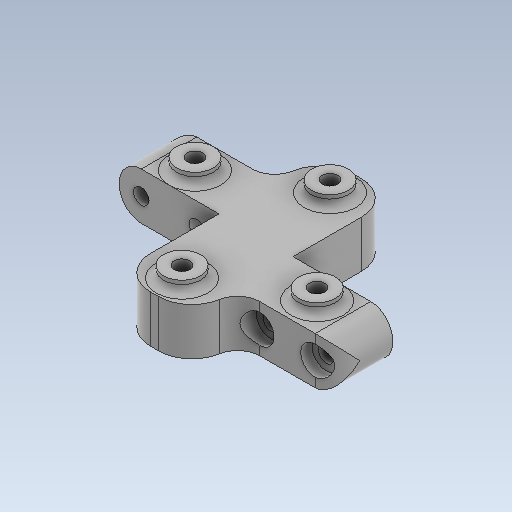
# Autodesk Inventor part: motor_mount
Saved by Autodesk Inventor 2021 (Build 250183000, 183)
## iProperties
Created: 2021-01-21
Part Number: motor_mount
Material: PC/ABS 플라스틱
Document SubType Name: Modeling
Designer: leejun
Density: 0.357273 g/cm^3
Appearance: 매끄러움 - 중간 회색
Author: leejun
Autodesk Inventor part; units mm, degrees
ref_plane "YZ Plane" through (0, 0, 0) normal (1, 0, 0) x (0, 1, 0)
ref_plane "XZ Plane" through (0, 0, 0) normal (0, 1, 0) x (-1, 0, 0)
ref_plane "XY Plane" through (0, 0, 0) normal (0, 0, 1) x (1, 0, 0)
sketch "스케치1" plane through (0, 0, 0) normal (0, 1, 0) x (-1, 0, 0)
  line L0 (-90, -12.7) -> (-10, -12.7) construction
  line L1 (-10, -12.7) -> (-10, 0) construction
  line L2 (-10, 0) -> (-90, 0) construction
  line L3 (-90, 0) -> (-90, -12.7) construction
  line L4 (10, 0) -> (90, 0) construction
  line L5 (90, 0) -> (90, 12.7) construction
  line L6 (90, 12.7) -> (10, 12.7) construction
  line L7 (10, 12.7) -> (10, 0) construction
  line L8 (126, 0) -> (-126, 0) projected
  line L9 (0, -38.5) -> (0, 38.5) projected
  line L10 (-37, 15) -> (10, 15)
  line L11 (10, 15) -> (10, 0)
  line L12 (10, 0) -> (-37, 0)
  line L13 (-37, 0) -> (-37, 15)
  line L14 (37, -15) -> (-10, -15)
  line L15 (-10, -15) -> (-10, 0)
  line L16 (-10, 0) -> (37, 0)
  line L17 (37, 0) -> (37, -15)
  line L18 (-10, -27.5) -> (10, -27.5)
  line L19 (10, -27.5) -> (10, 27.5)
  line L20 (10, 27.5) -> (-10, 27.5)
  line L21 (-10, 27.5) -> (-10, -27.5)
  point P0 (10, 15)
  point P1 (-10, 15)
  point P2 (-37, 0)
  point P3 (10, -15)
  point P4 (37, 0)
  dimension "d68" = 12.7
  dimension "d69" = 80
  dimension "d70" = 20
  dimension "d71" = 27
  dimension "d72" = 15
  dimension "d73" = 55
  constraints: 40 end point, 14 parallel, 7 collinear, 5 perpendicular, 4 horizontal, 3 other
  measures "d68" distance of L0.end L1.end
  measures "d69" distance of L0.start L0.end
  measures "d70" distance between parallel lines of L7 L1
  measures "d71" distance between parallel lines of L17 L7
  measures "d72" distance of L16.end L14.start
  measures "d73" distance of L18.end L19.end
extrude "돌출1" add sketch "스케치1" along normal blind 12.7
sketch "스케치5" plane through (37, 0, 0) normal (0, 0, -1) x (-1, 0, 0)
  line L0 (0, 0) -> (27, 0) projected
  line L1 (27, 0) -> (27, 12.7) projected
  line L2 (0, 12.7) -> (27, 12.7) projected
  line L3 (0, 0) -> (0, 12.7) projected
  circle A0 centre (6, 6.35) radius 6.35
  circle A1 centre (21, 6.35) radius 2.1
  circle A2 centre (6, 6.35) radius 2.1
  line L4 (0, 0) -> (27, 0) projected
  point P0 (37, 0)
  dimension "d74" = 4.2
  dimension "d75" = 6
  dimension "d76" = 15
  constraints: 3 centre point, 2 tangent, 1 coincident, 1 equal radius, 1 horizontal alignment
  measures "d74" diameter of A2
  measures "d75" distance from line of L1 A1.centre
  measures "d76" distance of A1.centre A0.centre
extrude "돌출6" cut sketch "스케치5" against normal through all contours A1 | A2
sketch "스케치6" plane through (10, 0, 15) normal (0, 0, 1) x (1, 0, 0)
  circle A0 centre (6, 6.35) radius 2.1 projected
  circle A1 centre (21, 6.35) radius 2.1 projected
  line L0 (0, 0) -> (27, 0) projected
  line L1 (27, 0) -> (27, 12.7) projected
  line L2 (0, 12.7) -> (27, 12.7) projected
  line L3 (0, 0) -> (0, 12.7) projected
  circle A2 centre (6, 6.35) radius 3.9
  circle A3 centre (21, 6.35) radius 3.9
  point P0 (-10, 0)
  dimension "d82" = 7.8
  constraints: 2 centre point, 2 coincident, 1 equal radius
  measures "d82" diameter of A2
extrude "돌출7" cut sketch "스케치6" against normal blind 3 contours A2 | A3
pattern_circular "원형 패턴3" count 2 over 360 about axis through (0, -10, 0) along (0, 1, 0) of "돌출6", "돌출7"
sketch "스케치7" plane through (0, 12.7, 0) normal (0, 1, 0) x (1, 0, 0)
  line L0 (13.9, -12) -> (18.1, -12) projected
  line L1 (13.9, 0) -> (18.1, 0) projected
  line L2 (28.9, -12) -> (33.1, -12) projected
  line L3 (28.9, 0) -> (33.1, 0) projected
  line L4 (-18.1, 12) -> (-13.9, 12) projected
  line L5 (-13.9, 0) -> (-18.1, 0) projected
  line L6 (-19.9, 12) -> (-12.1, 12) projected
  line L7 (-19.9, 15) -> (-12.1, 15) projected
  line L8 (-33.1, 12) -> (-28.9, 12) projected
  line L9 (-28.9, 0) -> (-33.1, 0) projected
  line L10 (-34.9, 12) -> (-27.1, 12) projected
  line L11 (-34.9, 15) -> (-27.1, 15) projected
  line L12 (19.9, -12) -> (12.1, -12) projected
  line L13 (19.9, -15) -> (12.1, -15) projected
  line L14 (34.9, -12) -> (27.1, -12) projected
  line L15 (34.9, -15) -> (27.1, -15) projected
  line L16 (19.9, -15) -> (12.1, -15) projected
  line L17 (12.1, -15) -> (12.1, -12)
  line L18 (13.9, 0) -> (18.1, 0) projected
  line L19 (13.9, 0) -> (13.9, -12)
  line L20 (13.9, 0) -> (13.9, -12) projected
  line L21 (18.1, 0) -> (18.1, -12)
  line L22 (18.1, 0) -> (18.1, -12) projected
  line L23 (19.9, -12) -> (12.1, -12) projected
  line L24 (19.9, -12) -> (19.9, -15)
  line L25 (19.9, -15) -> (19.9, -12) projected
  line L26 (34.9, -15) -> (27.1, -15) projected
  line L27 (27.1, -15) -> (27.1, -12)
  line L28 (27.1, -15) -> (27.1, -12) projected
  line L29 (34.9, -12) -> (27.1, -12) projected
  line L30 (34.9, -12) -> (34.9, -15)
  line L31 (34.9, -15) -> (34.9, -12) projected
  line L32 (28.9, -12) -> (33.1, -12) projected
  line L33 (28.9, 0) -> (28.9, -12)
  line L34 (33.1, 0) -> (33.1, -12)
  line L35 (37, 0) -> (10, 0) projected
  line L36 (-13.9, 0) -> (-18.1, 0) projected
  line L37 (-18.1, 0) -> (-18.1, 12)
  line L38 (-18.1, 0) -> (-18.1, 12) projected
  line L39 (-19.9, 12) -> (-12.1, 12) projected
  line L40 (-19.9, 12) -> (-19.9, 15)
  line L41 (-19.9, 15) -> (-19.9, 12) projected
  line L42 (-12.1, 15) -> (-12.1, 12)
  line L43 (-12.1, 15) -> (-12.1, 12) projected
  line L44 (-13.9, 0) -> (-13.9, 12)
  line L45 (-13.9, 0) -> (-13.9, 12) projected
  line L46 (-33.1, 12) -> (-28.9, 12) projected
  line L47 (-28.9, 0) -> (-28.9, 12)
  line L48 (-33.1, 0) -> (-33.1, 12)
  line L49 (-37, 0) -> (-10, 0) projected
  line L50 (-34.9, 12) -> (-34.9, 15)
  line L51 (-27.1, 15) -> (-27.1, 12)
  line L52 (-27.1, 15) -> (-27.1, 12) projected
  line L53 (-10, -27.5) -> (10, -27.5) projected
  line L54 (10, -27.5) -> (10, -15) projected
  line L55 (10, -15) -> (37, -15) projected
  line L56 (37, -15) -> (37, 0) projected
  line L57 (37, 0) -> (10, 0) projected
  line L58 (10, 0) -> (10, 27.5) projected
  line L59 (10, 27.5) -> (-10, 27.5) projected
  line L60 (-10, 27.5) -> (-10, 15) projected
  line L61 (-10, 15) -> (-37, 15) projected
  line L62 (-37, 15) -> (-37, 0) projected
  line L63 (-37, 0) -> (-10, 0) projected
  line L64 (-10, 0) -> (-10, -27.5) projected
  circle A0 centre (0, -20) radius 2.1
  circle A1 centre (0, 20) radius 2.1
  circle A2 centre (23.5, -7) radius 2.1
  circle A3 centre (-23.5, 7) radius 2.1
  line L65 (0, 38.5) -> (0, -38.5) projected
  line L66 (-51.8, 0) -> (51.8, 0) projected
  line L67 (23.5, -7) -> (-23.5, -7) construction
  line L68 (-23.5, -7) -> (-23.5, 7) construction
  line L69 (-23.5, 7) -> (23.5, 7) construction
  line L70 (23.5, 7) -> (23.5, -7) construction
  point P0 (0, 0)
  dimension "d85" = 4.2
  dimension "d86" = 20
  dimension "d87" = 5.4
  dimension "d88" = 5.4
  dimension "d89" = 7
  constraints: 40 end point, 10 collinear, 4 centre point, 4 equal radius, 4 parallel, 4 perpendicular, 2 vertical, 1 horizontal, 1 point on line, 2 other
  measures "d85" diameter of A3
  measures "d87" distance between parallel lines of L21 L70
  measures "d88" distance between parallel lines of L33 L70
  measures "d89" distance of the line from the sketch origin of L67
extrude "돌출8" cut sketch "스케치7" against normal through all contours L65 A1 | A1 L65 | L65 A0 | A0 L65 | A2 | A3
fillet "모깎기4" radius 6 4 edges at (37, 6.35, 15) (10, 6.35, 15) (-10, 6.35, -15) (-37, 6.35, -15)
fillet "모깎기4" radius 9 4 edges at (-10, 6.35, -27.5) (10, 6.35, -27.5) (10, 6.35, 27.5) (-10, 6.35, 27.5)
sketch "스케치8" plane through (0, 12.7, 0) normal (0, 1, 0) x (1, 0, 0)
  arc A0 (-31, 15) -> (-37, 9) centre (-31, 9) ccw projected
  line L0 (-37, 9) -> (-37, 0) projected
  line L1 (-37, 0) -> (-10, 0) projected
  line L2 (-10, 0) -> (-10, -18.5) projected
  arc A1 (-10, -18.5) -> (-1, -27.5) centre (-1, -18.5) ccw projected
  line L3 (-1, -27.5) -> (1.2098, -27.5) projected
  arc A2 (1.2098, -27.5) -> (10.0839, -20) centre (1.2098, -18.5) ccw projected
  arc A3 (16, -15) -> (10.0839, -20) centre (16, -21) ccw projected
  line L4 (16, -15) -> (31, -15) projected
  arc A4 (31, -15) -> (37, -9) centre (31, -9) ccw projected
  line L5 (37, -9) -> (37, 0) projected
  line L6 (37, 0) -> (10, 0) projected
  line L7 (10, 0) -> (10, 18.5) projected
  arc A5 (10, 18.5) -> (1, 27.5) centre (1, 18.5) ccw projected
  line L8 (1, 27.5) -> (-1.2098, 27.5) projected
  arc A6 (-1.2098, 27.5) -> (-10.0839, 20) centre (-1.2098, 18.5) ccw projected
  arc A7 (-16, 15) -> (-10.0839, 20) centre (-16, 21) ccw projected
  line L9 (-16, 15) -> (-31, 15) projected
  circle A8 centre (23.5, -7) radius 2.1 projected
  circle A9 centre (0, -20) radius 2.1 projected
  circle A10 centre (0, 20) radius 2.1 projected
  circle A11 centre (-23.5, 7) radius 2.1 projected
  circle A12 centre (23.5, -7) radius 5
  circle A13 centre (0, -20) radius 5
  circle A14 centre (0, 20) radius 5
  circle A15 centre (-23.5, 7) radius 5
  point P0 (0, 0)
  dimension "d93" = 10
  constraints: 4 centre point, 4 coincident, 3 equal radius
  measures "d93" diameter of A12
extrude "돌출9" add sketch "스케치8" along normal blind 3 contours A12 | A13 | A14 | A15
sketch "스케치10" plane through (37, 0, 0) normal (0, 0, -1) x (-1, 0, 0)
  circle A0 centre (21, 6.35) radius 2.1 projected
  circle A1 centre (6, 6.35) radius 2.1 projected
  line L0 (0, 0) -> (27, 0) projected
  line L1 (27, 0) -> (27, 12.7) projected
  line L2 (0, 12.7) -> (27, 12.7) projected
  line L3 (0, 0) -> (0, 12.7) projected
  circle A2 centre (6, 6.35) radius 2.1 projected
  ellipse E0 centre (6, 6.35) end of major axis (0, 6.35) minor radius 6.35
  point P0 (37, 0)
  point P1 (6, 0)
  point P2 (0, 6.35)
  point P3 (6, 12.7)
  dimension "d103" = 6
  dimension "d102" = 6
  constraints: 1 coincident, 1 horizontal, 1 vertical, 2 other
  measures "d102" distance from line of A1.centre L3
extrude "돌출11" cut sketch "스케치10" against normal through all contours L3 E0 L0 | L3 L2 E0
pattern_circular "원형 패턴4" count 2 over 360 about axis through (0, -10, 0) along (0, 1, 0) of "돌출11"
fillet "모깎기8" radius 2 4 edges at (18.5, 12.7, 7) (-5, 12.7, 20) (-5, 12.7, -20) (-28.5, 12.7, -7)
